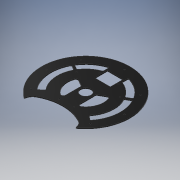
# Autodesk Inventor part: 3rdPlate
Saved by Autodesk Inventor 2017 (Build 210142000, 142)
## iProperties
Created: 2019-03-15
Part Number: 3rdPlate
Material: Generic
Document SubType Name: Modeling
Designer: Nicholas Cresswell
Density: 1 g/cm^3
Appearance: Smooth - Black
Author: Nicholas Cresswell
Autodesk Inventor part; units mm, degrees
ref_plane "YZ Plane" through (0, 0, 0) normal (1, 0, 0) x (0, 1, 0)
ref_plane "XZ Plane" through (0, 0, 0) normal (0, 1, 0) x (-1, 0, 0)
ref_plane "XY Plane" through (0, 0, 0) normal (0, 0, 1) x (1, 0, 0)
sketch "Sketch1" plane through (0, 0, 0) normal (0, 0, 1) x (1, 0, 0)
  circle A0 centre (22.4968, 30.1412) radius 1.5 projected
  circle A1 centre (-22.5032, 30.1412) radius 1.5 projected
  arc A2 (60.7504, -108.8306) -> (62.339, -109.5339) centre (61.7453, -108.7292) ccw projected
  arc A3 (60.7504, -108.8306) -> (50.0022, -92.7062) centre (40.1313, -110.9304) ccw projected
  arc A4 (50.0022, -92.7062) -> (-50.001, -92.7085) centre (0.0027, -185.0388) ccw projected
  arc A5 (-50.001, -92.7085) -> (-60.7494, -108.8311) centre (-40.1315, -110.9322) ccw projected
  arc A6 (-62.3379, -109.5344) -> (-60.7494, -108.8311) centre (-61.7442, -108.7297) ccw projected
  arc A7 (62.339, -109.5339) -> (-62.3379, -109.5344) centre (0.0002, -25.0416) ccw projected
  arc A8 (-40.7535, -11.3119) -> (-25.4619, -59.6998) centre (-0.0033, -25.0441) ccw projected
  arc A9 (-25.4619, -59.6998) -> (-17.5017, -55.6702) centre (-22.5017, -55.6702) ccw projected
  line L0 (-17.5017, -55.6702) -> (-17.5016, -25.0441) projected
  arc A10 (-17.2066, -21.8442) -> (-17.5016, -25.0441) centre (-0.0033, -25.0441) ccw projected
  arc A11 (-17.2066, -21.8442) -> (-19.6222, -16.5997) centre (-22.1222, -20.9298) ccw projected
  line L1 (-19.6222, -16.5997) -> (-33.5153, -8.5785) projected
  arc A12 (-33.5153, -8.5785) -> (-40.7535, -11.3119) centre (-36.0153, -12.9086) ccw projected
  line L2 (33.5098, -8.5818) -> (19.6211, -16.6006) projected
  arc A13 (19.6211, -16.6006) -> (17.2054, -21.8447) centre (22.1212, -20.9307) ccw projected
  arc A14 (17.5003, -25.0442) -> (17.2054, -21.8447) centre (-0.0033, -25.0441) ccw projected
  line L3 (17.5003, -25.0442) -> (17.5003, -55.6665) projected
  arc A15 (17.5003, -55.6665) -> (25.4611, -59.6955) centre (22.5003, -55.6665) ccw projected
  arc A16 (25.4611, -59.6955) -> (40.7482, -11.3157) centre (-0.0033, -25.0441) ccw projected
  arc A17 (40.7482, -11.3157) -> (33.5098, -8.5818) centre (36.0099, -12.9119) ccw projected
  arc A18 (-25.1118, 53.5439) -> (-69.0324, 20.1388) centre (-0.0033, -25.0441) ccw
  arc A19 (-69.0324, 20.1388) -> (-68.359, 17.3114) centre (-67.359, 19.0434) ccw projected
  line L4 (-68.359, 17.3114) -> (-58.789, 11.7862) projected
  arc A20 (-58.789, 11.7862) -> (-56.1254, 12.408) centre (-57.789, 13.5182) ccw projected
  arc A21 (-23.7978, 38.0921) -> (-56.1254, 12.408) centre (-0.0033, -25.0441) ccw
  arc A22 (-73.7424, -55.6421) -> (-75.5895, -54.9212) centre (-75.6955, -57.9193) ccw projected
  arc A23 (-73.7424, -55.6421) -> (-71.4404, -55.8561) centre (-72.4403, -54.124) ccw projected
  line L5 (-71.4404, -55.8561) -> (-63.925, -51.5171) projected
  arc A24 (-63.925, -51.5171) -> (-63.0561, -49.0729) centre (-64.925, -49.7851) ccw projected
  arc A25 (-60.5006, 4.8409) -> (-63.0561, -49.0729) centre (-0.0033, -25.0441) ccw projected
  arc A26 (-60.5006, 4.8409) -> (-61.2937, 7.4588) centre (-62.2937, 5.7267) ccw projected
  line L6 (-61.2937, 7.4588) -> (-70.8555, 12.9792) projected
  arc A27 (-70.8555, 12.9792) -> (-73.6407, 12.1489) centre (-71.8555, 11.2472) ccw projected
  arc A28 (-73.6407, 12.1489) -> (-77.3951, -53.6151) centre (-0.0033, -25.0441) ccw projected
  arc A29 (-77.3951, -53.6151) -> (-75.5895, -54.9212) centre (-75.5189, -52.9224) ccw projected
  arc A30 (56.1187, 12.4083) -> (58.7823, 11.7864) centre (57.7823, 13.5184) ccw projected
  line L7 (58.7823, 11.7864) -> (68.3445, 17.3071) projected
  arc A31 (68.3445, 17.3071) -> (69.0178, 20.1345) centre (67.3445, 19.0391) ccw projected
  arc A32 (69.0178, 20.1345) -> (25.1056, 53.5343) centre (-0.0033, -25.0441) ccw
  arc A33 (77.3822, -53.6189) -> (73.6301, 12.1465) centre (-0.0033, -25.0441) ccw projected
  arc A34 (73.6301, 12.1465) -> (70.8449, 12.9769) centre (71.8449, 11.2448) ccw projected
  line L8 (70.8449, 12.9769) -> (61.29, 7.4604) projected
  arc A35 (61.29, 7.4604) -> (60.4969, 4.8425) centre (62.29, 5.7283) ccw projected
  arc A36 (63.0533, -49.0722) -> (60.4969, 4.8425) centre (-0.0033, -25.0441) ccw projected
  arc A37 (63.0533, -49.0722) -> (63.9222, -51.5164) centre (64.9222, -49.7844) ccw projected
  line L9 (63.9222, -51.5164) -> (71.4454, -55.86) projected
  arc A38 (71.4454, -55.86) -> (73.7479, -55.6457) centre (72.4454, -54.1279) ccw projected
  arc A39 (75.5842, -54.9246) -> (73.7479, -55.6457) centre (75.7016, -57.9223) ccw projected
  arc A40 (75.5842, -54.9246) -> (77.3822, -53.6189) centre (75.506, -52.9261) ccw projected
  circle A41 centre (0, -25.0414) radius 12.5 projected
  arc A42 (63.3702, -73.6036) -> (63.6677, -75.5605) centre (66.3188, -74.1564) ccw projected
  arc A43 (63.3702, -73.6036) -> (62.4045, -71.503) centre (61.4045, -73.235) ccw projected
  line L10 (62.4045, -71.503) -> (54.8893, -67.1641) projected
  arc A44 (54.8893, -67.1641) -> (52.3379, -67.6338) centre (53.8893, -68.8961) ccw projected
  arc A45 (42.3269, -77.5955) -> (52.3379, -67.6338) centre (-0.0033, -25.0441) ccw projected
  arc A46 (42.3269, -77.5955) -> (42.8203, -81.0025) centre (43.5815, -79.153) ccw projected
  arc A47 (53.5093, -86.0748) -> (42.8203, -81.0025) centre (0.0002, -185.037) ccw projected
  arc A48 (53.5093, -86.0748) -> (55.8138, -85.7882) centre (54.4606, -84.3155) ccw projected
  arc A49 (55.8138, -85.7882) -> (63.4384, -77.775) centre (-0.0033, -25.0441) ccw projected
  arc A50 (63.4384, -77.775) -> (63.6677, -75.5605) centre (61.9003, -76.4966) ccw projected
  arc A51 (-63.444, -77.7749) -> (-55.8167, -85.7905) centre (-0.0033, -25.0441) ccw projected
  arc A52 (-55.8167, -85.7905) -> (-53.5122, -86.077) centre (-54.4635, -84.3178) ccw projected
  arc A53 (-42.8207, -81.0032) -> (-53.5122, -86.077) centre (0.0002, -185.037) ccw projected
  arc A54 (-42.8207, -81.0032) -> (-42.3274, -77.5961) centre (-43.5819, -79.1538) ccw projected
  arc A55 (-52.3409, -67.6331) -> (-42.3274, -77.5961) centre (-0.0033, -25.0441) ccw projected
  arc A56 (-52.3409, -67.6331) -> (-54.8922, -67.1633) centre (-53.8922, -68.8954) ccw projected
  line L11 (-54.8922, -67.1633) -> (-62.4125, -71.5052) projected
  arc A57 (-62.4125, -71.5052) -> (-63.3781, -73.6065) centre (-61.4125, -73.2373) ccw projected
  arc A58 (-63.6742, -75.562) -> (-63.3781, -73.6065) centre (-66.3266, -74.1603) ccw projected
  arc A59 (-63.6742, -75.562) -> (-63.444, -77.7749) centre (-61.9059, -76.4965) ccw projected
  line L12 (-22.5032, 51.6387) -> (-22.5032, 39.9636)
  line L13 (22.4968, 39.9635) -> (22.4968, 51.6291)
  arc A60 (56.1187, 12.4083) -> (23.7915, 38.092) centre (-0.0033, -25.0441) ccw
  arc A61 (25.1056, 53.5343) -> (22.4968, 51.6291) centre (24.4968, 51.6291) ccw
  arc A62 (22.4968, 39.9635) -> (23.7915, 38.092) centre (24.4968, 39.9635) ccw
  arc A63 (-23.7978, 38.0921) -> (-22.5032, 39.9636) centre (-24.5032, 39.9636) ccw
  arc A64 (-22.5032, 51.6387) -> (-25.1118, 53.5439) centre (-24.5032, 51.6387) ccw
  line L14 (17.4968, 44.3912) -> (17.4968, 45.3912) construction
  line L15 (17.4968, 44.3912) -> (18.4968, 44.3912) construction
  line L16 (18.4968, 44.3912) -> (18.4968, 45.3912) construction
  line L17 (18.4968, 45.3912) -> (17.4968, 45.3912) construction
  line L18 (-17.5032, 15.8912) -> (-17.5032, 14.8912) construction
  line L19 (-17.5032, 14.8912) -> (-18.5032, 14.8912) construction
  line L20 (18.4968, 45.3912) -> (-18.5032, 45.3912)
  line L21 (-18.5032, 45.3912) -> (-18.5032, 14.8912)
  line L22 (-18.5032, 14.8912) -> (18.4968, 14.8912)
  line L23 (18.4968, 14.8912) -> (18.4968, 45.3912)
  point P0 (0, 0)
  point P1 (-22.5032, 54.3301)
  point P2 (-17.5032, 40.1181)
  point P3 (22.4968, 54.3206)
  point P4 (22.4968, 38.5649)
  point P5 (-22.5032, 38.565)
  dimension "d4" = 2
  dimension "d9" = 1
  dimension "d10" = 1
  dimension "d11" = 1
  dimension "d12" = 1
  constraints: 24 end point, 20 point on circle, 8 centre point, 8 tangent, 4 perpendicular, 4 point on line, 3 equal radius, 2 parallel, 1 horizontal, 1 vertical
  measures "d4" radius of A61
  measures "d9" distance of L14.start L14.end
  measures "d10" distance of L14.start L15.end
  measures "d11" distance of L18.start L18.end
  measures "d12" distance of L18.end L19.end
extrude "Extrusion5" add sketch "Sketch1" against normal blind 2
sketch "Sketch4" plane through (0, 0, -2) normal (0, 0, -1) x (-1, 0, 0)
  circle A0 centre (92.5005, -25.0414) radius 1.5 projected
  circle A1 centre (-92.4893, -25.0414) radius 1.5 projected
  point P0 (0, 0)
extrude "Extrusion6" cut sketch "Sketch4" against normal up to next
sketch "Sketch5" plane through (0, 0, -2) normal (0, 0, -1) x (-1, 0, 0)
  circle A0 centre (0, -25.0414) radius 12.5 projected
  line L0 (0, -25.0414) -> (70.8591, -84.4992) construction
  line L1 (0, -25.0414) -> (92.5, -25.0414) construction
  circle A1 centre (70.8591, -84.4992) radius 1.5
  line L2 (0, -25.0414) -> (-70.8591, -84.4992) construction
  line L3 (0, -25.0414) -> (92.5, -25.0414) construction
  circle A2 centre (-70.8591, -84.4992) radius 1.5
  line L4 (0, -25.0414) -> (-70.8591, 34.4165) construction
  line L5 (0, -25.0414) -> (92.5, -25.0414) construction
  line L6 (0, -25.0414) -> (70.8591, 34.4165) construction
  line L7 (0, -25.0414) -> (92.5, -25.0414) construction
  circle A3 centre (-70.8591, 34.4165) radius 1.5
  circle A4 centre (70.8591, 34.4165) radius 1.5
  circle A5 centre (0, 67.4586) radius 1.5
  line L8 (0, 67.4586) -> (0, -25.0414) construction
  line L9 (68.359, 17.3114) -> (58.789, 11.7862) construction
  line L10 (61.2937, 7.4588) -> (70.8555, 12.9792) construction
  arc A6 (56.1254, 12.408) -> (58.789, 11.7862) centre (57.789, 13.5182) ccw construction
  arc A7 (61.2937, 7.4588) -> (60.5006, 4.8409) centre (62.2937, 5.7267) ccw construction
  line L11 (56.1254, 12.408) -> (60.5006, 4.8409) construction
  line L12 (58.313, 8.6245) -> (51.8178, 4.8745) construction
  line L13 (58.313, 8.6245) -> (65.813, 8.6245) construction
  circle A8 centre (51.8178, 4.8745) radius 1.5
  line L14 (-56.1255, 12.408) -> (-60.5006, 4.8409) construction
  line L15 (-58.313, 8.6245) -> (-51.8178, 4.8745) construction
  circle A9 centre (-51.8178, 4.8745) radius 1.5
  point P0 (0, 0)
  dimension "d18" = 92.5
  dimension "d19" = 40
  dimension "d20" = 3
  dimension "d21" = 92.5
  dimension "d22" = 140
  dimension "d23" = 3
  dimension "d24" = 92.5
  dimension "d25" = 140
  dimension "d26" = 92.5
  dimension "d27" = 40
  dimension "d28" = 3
  dimension "d29" = 3
  dimension "d31" = 3
  dimension "d32" = 92.5
  dimension "d33" = 7.5
  dimension "d34" = 150
  dimension "d35" = 3
  constraints: 28 end point, 7 centre point, 6 coincident, 5 equal length, 5 horizontal, 5 symmetric about line, 1 midpoint, 1 perpendicular, 1 other
  measures "d18" distance of L0.start L0.end
  measures "d19" angle of L0 L1
  measures "d20" diameter of A1
  measures "d21" distance of L0.start L2.end
  measures "d22" angle of L2 L3
  measures "d23" diameter of A2
  measures "d24" distance of L0.start L4.end
  measures "d25" angle of L5 L4
  measures "d26" distance of L0.start L6.end
  measures "d27" angle of L7 L6
  measures "d28" diameter of A3
  measures "d29" diameter of A4
  measures "d31" diameter of A5
  measures "d32" distance of L8.start L0.start
  measures "d33" distance of L12.start L12.end
  measures "d34" angle of L12 L13
  measures "d35" diameter of A8
extrude "Extrusion7" cut sketch "Sketch5" against normal up to next contours A1 | A2 | A3 | A4 | A5 | A8 | A9
sketch "Sketch6" plane through (0, 0, -2) normal (0, 0, -1) x (-1, 0, 0)
  line L0 (-17.5003, -25.0442) -> (-17.5003, -55.6665) construction
  line L1 (-17.5003, -55.6665) -> (-17.5003, -94.1691) construction
  arc A0 (17.5017, -55.6702) -> (25.4619, -59.6998) centre (22.5017, -55.6702) ccw projected
  line L2 (17.5017, -55.6702) -> (17.5017, -94.1691) construction
  arc A1 (-42.8203, -81.0025) -> (-42.3269, -77.5955) centre (-43.5815, -79.153) ccw construction
  line L3 (-42.8203, -81.0025) -> (-17.5003, -70.5922) construction
  line L4 (-42.8203, -81.0025) -> (-15.4437, -81.0025) construction
  arc A2 (53.5122, -86.077) -> (42.8207, -81.0032) centre (-0.0002, -185.037) ccw construction
  arc A3 (42.3274, -77.5961) -> (42.8207, -81.0032) centre (43.5819, -79.1538) ccw construction
  circle A4 centre (-17.5003, -70.5922) radius 1.5
  line L5 (-17.5003, -70.5922) -> (17.5017, -70.5922)
  line L6 (17.5017, -70.5922) -> (42.8207, -81.0032) construction
  circle A5 centre (17.5017, -70.5922) radius 1.5
  point P0 (0, 0)
  dimension "d38" = 22.35
  dimension "d39" = 3
  dimension "d40" = 3
  constraints: 12 end point, 2 centre point, 2 coincident, 2 point on line, 2 vertical, 1 equal length, 1 horizontal, 1 perpendicular, 1 tangent
  measures "d38" angle of L4 L3
  measures "d39" diameter of A4
  measures "d40" diameter of A5
extrude "Extrusion8" cut sketch "Sketch6" against normal up to next
sketch "Sketch8" plane through (0, 0, 0) normal (0, 0, 1) x (1, 0, 0)
  line L0 (54.8893, -67.1641) -> (62.4045, -71.503) projected
  arc A0 (42.3269, -77.5955) -> (52.3379, -67.6338) centre (-0.0033, -25.0441) ccw projected
  arc A1 (54.8893, -67.1641) -> (52.3379, -67.6338) centre (53.8893, -68.8961) ccw projected
  arc A2 (63.3702, -73.6036) -> (62.4045, -71.503) centre (61.4045, -73.235) ccw projected
  arc A3 (63.3702, -73.6036) -> (63.6677, -75.5605) centre (66.3188, -74.1564) ccw projected
  arc A4 (63.4384, -77.775) -> (63.6677, -75.5605) centre (61.9003, -76.4966) ccw projected
  arc A5 (55.8138, -85.7882) -> (63.4384, -77.775) centre (-0.0033, -25.0441) ccw projected
  arc A6 (53.5093, -86.0748) -> (55.8138, -85.7882) centre (54.4606, -84.3155) ccw projected
  arc A7 (53.5093, -86.0748) -> (42.8203, -81.0025) centre (0.0002, -185.037) ccw projected
  arc A8 (42.3269, -77.5955) -> (42.8203, -81.0025) centre (43.5815, -79.153) ccw projected
  arc A9 (-63.6742, -75.562) -> (-63.3781, -73.6065) centre (-66.3266, -74.1603) ccw projected
  arc A10 (-62.4125, -71.5052) -> (-63.3781, -73.6065) centre (-61.4125, -73.2373) ccw projected
  line L1 (-62.4125, -71.5052) -> (-54.8922, -67.1633) projected
  arc A11 (-52.3409, -67.6331) -> (-54.8922, -67.1633) centre (-53.8922, -68.8954) ccw projected
  arc A12 (-52.3409, -67.6331) -> (-42.3274, -77.5961) centre (-0.0033, -25.0441) ccw projected
  arc A13 (-42.8207, -81.0032) -> (-42.3274, -77.5961) centre (-43.5819, -79.1538) ccw projected
  arc A14 (-42.8207, -81.0032) -> (-53.5122, -86.077) centre (0.0002, -185.037) ccw projected
  arc A15 (-55.8167, -85.7905) -> (-53.5122, -86.077) centre (-54.4635, -84.3178) ccw projected
  arc A16 (-63.444, -77.7749) -> (-55.8167, -85.7905) centre (-0.0033, -25.0441) ccw projected
  arc A17 (-63.6742, -75.562) -> (-63.444, -77.7749) centre (-61.9059, -76.4965) ccw projected
  point P0 (0, 0)
extrude "Extrusion9" add sketch "Sketch8" against normal blind 2
sketch "Sketch9" plane through (0, 0, 0) normal (0, 0, 1) x (1, 0, 0)
  circle A0 centre (0, -25.0414) radius 12.5 construction
  arc A1 (51.6905, -68.4148) -> (60.462, 4.9171) centre (0, -25.0414) ccw construction
  circle A2 centre (70.8591, -84.4992) radius 1.5 construction
  line L0 (0, -25.0414) -> (61.6386, -76.7623) construction
  circle A3 centre (-70.8591, -84.4992) radius 1.5 construction
  line L1 (-61.6386, -76.7623) -> (0, -25.0414) construction
  arc A4 (61.29, 7.4604) -> (60.4969, 4.8425) centre (62.29, 5.7283) ccw
  line L2 (61.29, 7.4604) -> (70.8449, 12.9769)
  arc A5 (73.6301, 12.1465) -> (70.8449, 12.9769) centre (71.8449, 11.2448) ccw
  line L3 (-70.8555, 12.9792) -> (-61.2938, 7.4587)
  arc A6 (-60.5006, 4.8409) -> (-61.2938, 7.4587) centre (-62.2938, 5.7267) ccw
  arc A7 (-70.8555, 12.9792) -> (-73.6407, 12.1488) centre (-71.8555, 11.2472) ccw
  arc A8 (-60.5005, 4.841) -> (-52.9182, -66.9094) centre (0, -25.0414) ccw
  arc A9 (52.9183, -66.9094) -> (60.4545, 4.9342) centre (0, -25.0414) ccw
  line L4 (-61.6386, -76.7623) -> (-53.2011, -69.6824)
  line L5 (53.2012, -69.6824) -> (61.6386, -76.7623)
  arc A10 (73.6301, 12.1465) -> (70.8449, 12.9769) centre (71.8449, 11.2448) ccw projected
  arc A11 (-73.5375, 12.3292) -> (-64.4878, -76.4774) centre (0, -25.0414) ccw
  arc A12 (77.3822, -53.6189) -> (73.6301, 12.1465) centre (-0.0033, -25.0441) ccw projected
  arc A13 (64.4878, -76.4774) -> (73.6301, 12.1465) centre (0, -25.0414) ccw
  arc A14 (-64.4878, -76.4774) -> (-61.6386, -76.7623) centre (-62.9242, -75.2302) ccw
  arc A15 (-53.2011, -69.6824) -> (-52.9182, -66.9094) centre (-54.4867, -68.1504) ccw
  arc A16 (61.6386, -76.7623) -> (64.4878, -76.4774) centre (62.9242, -75.2302) ccw
  arc A17 (52.9183, -66.9094) -> (53.2012, -69.6824) centre (54.4867, -68.1504) ccw
  point P0 (0, 0)
  point P1 (-51.6911, -68.4154)
  point P2 (51.6911, -68.4154)
  point P3 (63.1898, -78.0639)
  point P4 (-63.1897, -78.0639)
  dimension "d45" = 2
  dimension "d46" = 2
  constraints: 36 point on circle, 13 centre point, 12 end point, 9 point on line, 8 tangent, 4 coincident, 2 equal radius, 1 collinear
  measures "d45" radius of A14
  measures "d46" radius of A16
extrude "Extrusion10" cut sketch "Sketch9" against normal blind 2
body "Solid3"
